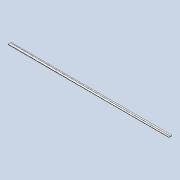
# Autodesk Inventor part: HTD 3M 780mm Open End Belt
Saved by Autodesk Inventor 2022 (Build 260153000, 153)
## iProperties
Created: 2021-10-10
Part Number: HTD 3M 780mm Open End Belt
Material: Generic
Document SubType Name: Modeling
Designer: Coy
Density: 1 g/cm^3
Appearance: Snow
Author: Coy
Autodesk Inventor part; units mm, degrees
(part 1 of 4)
ref_plane "YZ Plane" through (0, 0, 0) normal (1, 0, 0) x (0, 1, 0)
ref_plane "XZ Plane" through (0, 0, 0) normal (0, 1, 0) x (-1, 0, 0)
ref_plane "XY Plane" through (0, 0, 0) normal (0, 0, 1) x (1, 0, 0)
sketch "Sketch1" plane through (0, 0, 0) normal (0, 0, 1) x (1, 0, 0)
  line L0 (0, 2.4) -> (-3, 2.4)
  line L1 (0, 0) -> (-3, 0) construction
  line L2 (0, 2.4) -> (0, 0)
  line L3 (-3, 0) -> (-3, 2.4) construction
  arc A0 (-0.8878, 0.9525) -> (0, 0) centre (0, 0.89) ccw
  arc A1 (-3, 0) -> (-2.1122, 0.9525) centre (-3, 0.89) ccw
  line L4 (-1.1372, 1.22) -> (-1.8628, 1.22) construction
  line L5 (-1.5, 1.22) -> (-1.5, 0) construction
  line L6 (-1.8628, 1.22) -> (-1.1372, 1.22)
  arc A2 (-1.8628, 1.22) -> (-2.1122, 0.9525) centre (-1.8628, 0.97) ccw
  arc A3 (-0.8878, 0.9525) -> (-1.1372, 1.22) centre (-1.1372, 0.97) ccw
  line L7 (-6, 2.4) -> (-3, 2.4)
  line L8 (-6, 0) -> (-3, 0) construction
  line L9 (-6, 2.4) -> (-6, 0) construction
  arc A4 (-6, 0) -> (-5.1122, 0.9525) centre (-6, 0.89) ccw
  arc A5 (-3.8878, 0.9525) -> (-3, 0) centre (-3, 0.89) ccw
  line L10 (-4.8628, 1.22) -> (-4.1372, 1.22) construction
  line L11 (-4.5, 1.22) -> (-4.5, 0) construction
  line L12 (-4.1372, 1.22) -> (-4.8628, 1.22)
  arc A6 (-3.8878, 0.9525) -> (-4.1372, 1.22) centre (-4.1372, 0.97) ccw
  arc A7 (-4.8628, 1.22) -> (-5.1122, 0.9525) centre (-4.8628, 0.97) ccw
  line L13 (-12, 2.4) -> (-9, 2.4)
  line L14 (-12, 0) -> (-9, 0) construction
  line L15 (-12, 2.4) -> (-12, 0) construction
  line L16 (-9, 0) -> (-9, 2.4) construction
  arc A8 (-12, 0) -> (-11.1122, 0.9525) centre (-12, 0.89) ccw
  arc A9 (-9.8878, 0.9525) -> (-9, 0) centre (-9, 0.89) ccw
  line L17 (-10.8628, 1.22) -> (-10.1372, 1.22) construction
  line L18 (-10.5, 1.22) -> (-10.5, 0) construction
  line L19 (-10.1372, 1.22) -> (-10.8628, 1.22)
  arc A10 (-9.8878, 0.9525) -> (-10.1372, 1.22) centre (-10.1372, 0.97) ccw
  arc A11 (-10.8628, 1.22) -> (-11.1122, 0.9525) centre (-10.8628, 0.97) ccw
  line L20 (-6, 2.4) -> (-9, 2.4)
  line L21 (-6, 0) -> (-9, 0) construction
  arc A12 (-6.8878, 0.9525) -> (-6, 0) centre (-6, 0.89) ccw
  arc A13 (-9, 0) -> (-8.1122, 0.9525) centre (-9, 0.89) ccw
  line L22 (-7.1372, 1.22) -> (-7.8628, 1.22) construction
  line L23 (-7.5, 1.22) -> (-7.5, 0) construction
  line L24 (-7.8628, 1.22) -> (-7.1372, 1.22)
  arc A14 (-7.8628, 1.22) -> (-8.1122, 0.9525) centre (-7.8628, 0.97) ccw
  arc A15 (-6.8878, 0.9525) -> (-7.1372, 1.22) centre (-7.1372, 0.97) ccw
  line L25 (-24, 2.4) -> (-21, 2.4)
  line L26 (-24, 0) -> (-21, 0) construction
  line L27 (-24, 2.4) -> (-24, 0) construction
  line L28 (-21, 0) -> (-21, 2.4) construction
  arc A16 (-24, 0) -> (-23.1122, 0.9525) centre (-24, 0.89) ccw
  arc A17 (-21.8878, 0.9525) -> (-21, 0) centre (-21, 0.89) ccw
  line L29 (-22.8628, 1.22) -> (-22.1372, 1.22) construction
  line L30 (-22.5, 1.22) -> (-22.5, 0) construction
  line L31 (-22.1372, 1.22) -> (-22.8628, 1.22)
  arc A18 (-21.8878, 0.9525) -> (-22.1372, 1.22) centre (-22.1372, 0.97) ccw
  arc A19 (-22.8628, 1.22) -> (-23.1122, 0.9525) centre (-22.8628, 0.97) ccw
  line L32 (-18, 2.4) -> (-21, 2.4)
  line L33 (-18, 0) -> (-21, 0) construction
  line L34 (-18, 2.4) -> (-18, 0) construction
  arc A20 (-18.8878, 0.9525) -> (-18, 0) centre (-18, 0.89) ccw
  arc A21 (-21, 0) -> (-20.1122, 0.9525) centre (-21, 0.89) ccw
  line L35 (-19.1372, 1.22) -> (-19.8628, 1.22) construction
  line L36 (-19.5, 1.22) -> (-19.5, 0) construction
  line L37 (-19.8628, 1.22) -> (-19.1372, 1.22)
  arc A22 (-19.8628, 1.22) -> (-20.1122, 0.9525) centre (-19.8628, 0.97) ccw
  arc A23 (-18.8878, 0.9525) -> (-19.1372, 1.22) centre (-19.1372, 0.97) ccw
  line L38 (-15, 0) -> (-15, 2.4) construction
  arc A24 (-15.8878, 0.9525) -> (-15, 0) centre (-15, 0.89) ccw
  arc A25 (-15.8878, 0.9525) -> (-16.1372, 1.22) centre (-16.1372, 0.97) ccw
  line L39 (-16.5, 1.22) -> (-16.5, 0) construction
  line L40 (-16.8628, 1.22) -> (-16.1372, 1.22) construction
  line L41 (-16.1372, 1.22) -> (-16.8628, 1.22)
  arc A26 (-16.8628, 1.22) -> (-17.1122, 0.9525) centre (-16.8628, 0.97) ccw
  line L42 (-18, 0) -> (-15, 0) construction
  line L43 (-18, 2.4) -> (-15, 2.4)
  arc A27 (-18, 0) -> (-17.1122, 0.9525) centre (-18, 0.89) ccw
  line L44 (-12, 2.4) -> (-15, 2.4)
  line L45 (-12, 0) -> (-15, 0) construction
  arc A28 (-12.8878, 0.9525) -> (-12, 0) centre (-12, 0.89) ccw
  arc A29 (-15, 0) -> (-14.1122, 0.9525) centre (-15, 0.89) ccw
  line L46 (-13.1372, 1.22) -> (-13.8628, 1.22) construction
  arc A30 (-13.8628, 1.22) -> (-14.1122, 0.9525) centre (-13.8628, 0.97) ccw
  line L47 (-13.5, 1.22) -> (-13.5, 0) construction
  line L48 (-13.8628, 1.22) -> (-13.1372, 1.22)
  arc A31 (-12.8878, 0.9525) -> (-13.1372, 1.22) centre (-13.1372, 0.97) ccw
  line L49 (-48, 2.4) -> (-45, 2.4)
  line L50 (-48, 0) -> (-45, 0) construction
  line L51 (-48, 2.4) -> (-48, 0) construction
  line L52 (-45, 0) -> (-45, 2.4) construction
  arc A32 (-48, 0) -> (-47.1122, 0.9525) centre (-48, 0.89) ccw
  arc A33 (-45.8878, 0.9525) -> (-45, 0) centre (-45, 0.89) ccw
  line L53 (-46.8628, 1.22) -> (-46.1372, 1.22) construction
  line L54 (-46.5, 1.22) -> (-46.5, 0) construction
  line L55 (-46.1372, 1.22) -> (-46.8628, 1.22)
  arc A34 (-45.8878, 0.9525) -> (-46.1372, 1.22) centre (-46.1372, 0.97) ccw
  arc A35 (-46.8628, 1.22) -> (-47.1122, 0.9525) centre (-46.8628, 0.97) ccw
  line L56 (-42, 2.4) -> (-45, 2.4)
  line L57 (-42, 0) -> (-45, 0) construction
  line L58 (-42, 2.4) -> (-42, 0) construction
  arc A36 (-42.8878, 0.9525) -> (-42, 0) centre (-42, 0.89) ccw
  arc A37 (-45, 0) -> (-44.1122, 0.9525) centre (-45, 0.89) ccw
  line L59 (-43.1372, 1.22) -> (-43.8628, 1.22) construction
  line L60 (-43.5, 1.22) -> (-43.5, 0) construction
  line L61 (-43.8628, 1.22) -> (-43.1372, 1.22)
  arc A38 (-43.8628, 1.22) -> (-44.1122, 0.9525) centre (-43.8628, 0.97) ccw
  arc A39 (-42.8878, 0.9525) -> (-43.1372, 1.22) centre (-43.1372, 0.97) ccw
  line L62 (-39, 0) -> (-39, 2.4) construction
  arc A40 (-39.8878, 0.9525) -> (-39, 0) centre (-39, 0.89) ccw
  arc A41 (-39.8878, 0.9525) -> (-40.1372, 1.22) centre (-40.1372, 0.97) ccw
  line L63 (-40.5, 1.22) -> (-40.5, 0) construction
  line L64 (-40.8628, 1.22) -> (-40.1372, 1.22) construction
  line L65 (-40.1372, 1.22) -> (-40.8628, 1.22)
  arc A42 (-40.8628, 1.22) -> (-41.1122, 0.9525) centre (-40.8628, 0.97) ccw
  line L66 (-42, 0) -> (-39, 0) construction
  line L67 (-42, 2.4) -> (-39, 2.4)
  arc A43 (-42, 0) -> (-41.1122, 0.9525) centre (-42, 0.89) ccw
  line L68 (-36, 2.4) -> (-39, 2.4)
  line L69 (-36, 0) -> (-39, 0) construction
  line L70 (-36, 2.4) -> (-36, 0) construction
  arc A44 (-36.8878, 0.9525) -> (-36, 0) centre (-36, 0.89) ccw
  arc A45 (-39, 0) -> (-38.1122, 0.9525) centre (-39, 0.89) ccw
  line L71 (-37.1372, 1.22) -> (-37.8628, 1.22) construction
  arc A46 (-37.8628, 1.22) -> (-38.1122, 0.9525) centre (-37.8628, 0.97) ccw
  line L72 (-37.5, 1.22) -> (-37.5, 0) construction
  line L73 (-37.8628, 1.22) -> (-37.1372, 1.22)
  arc A47 (-36.8878, 0.9525) -> (-37.1372, 1.22) centre (-37.1372, 0.97) ccw
  line L74 (-27, 0) -> (-27, 2.4) construction
  arc A48 (-27.8878, 0.9525) -> (-27, 0) centre (-27, 0.89) ccw
  arc A49 (-27.8878, 0.9525) -> (-28.1372, 1.22) centre (-28.1372, 0.97) ccw
  line L75 (-28.5, 1.22) -> (-28.5, 0) construction
  line L76 (-28.8628, 1.22) -> (-28.1372, 1.22) construction
  line L77 (-28.1372, 1.22) -> (-28.8628, 1.22)
  arc A50 (-28.8628, 1.22) -> (-29.1122, 0.9525) centre (-28.8628, 0.97) ccw
  line L78 (-30, 0) -> (-27, 0) construction
  line L79 (-30, 2.4) -> (-27, 2.4)
  arc A51 (-30, 0) -> (-29.1122, 0.9525) centre (-30, 0.89) ccw
  line L80 (-30, 2.4) -> (-30, 0) construction
  arc A52 (-30.8878, 0.9525) -> (-30, 0) centre (-30, 0.89) ccw
  arc A53 (-30.8878, 0.9525) -> (-31.1372, 1.22) centre (-31.1372, 0.97) ccw
  line L81 (-31.5, 1.22) -> (-31.5, 0) construction
  line L82 (-31.1372, 1.22) -> (-31.8628, 1.22) construction
  line L83 (-31.8628, 1.22) -> (-31.1372, 1.22)
  arc A54 (-31.8628, 1.22) -> (-32.1122, 0.9525) centre (-31.8628, 0.97) ccw
  line L84 (-30, 0) -> (-33, 0) construction
  line L85 (-30, 2.4) -> (-33, 2.4)
  arc A55 (-33, 0) -> (-32.1122, 0.9525) centre (-33, 0.89) ccw
  line L86 (-33, 0) -> (-33, 2.4) construction
  arc A56 (-33.8878, 0.9525) -> (-33, 0) centre (-33, 0.89) ccw
  arc A57 (-33.8878, 0.9525) -> (-34.1372, 1.22) centre (-34.1372, 0.97) ccw
  line L87 (-34.5, 1.22) -> (-34.5, 0) construction
  line L88 (-34.8628, 1.22) -> (-34.1372, 1.22) construction
  line L89 (-34.1372, 1.22) -> (-34.8628, 1.22)
  arc A58 (-34.8628, 1.22) -> (-35.1122, 0.9525) centre (-34.8628, 0.97) ccw
  line L90 (-36, 2.4) -> (-33, 2.4)
  line L91 (-36, 0) -> (-33, 0) construction
  arc A59 (-36, 0) -> (-35.1122, 0.9525) centre (-36, 0.89) ccw
  line L92 (-24, 2.4) -> (-27, 2.4)
  line L93 (-24, 0) -> (-27, 0) construction
  arc A60 (-24.8878, 0.9525) -> (-24, 0) centre (-24, 0.89) ccw
  arc A61 (-27, 0) -> (-26.1122, 0.9525) centre (-27, 0.89) ccw
  arc A62 (-25.8628, 1.22) -> (-26.1122, 0.9525) centre (-25.8628, 0.97) ccw
  line L94 (-25.5, 1.22) -> (-25.5, 0) construction
  line L95 (-25.1372, 1.22) -> (-25.8628, 1.22) construction
  line L96 (-25.8628, 1.22) -> (-25.1372, 1.22)
  arc A63 (-24.8878, 0.9525) -> (-25.1372, 1.22) centre (-25.1372, 0.97) ccw
  line L97 (-96, 2.4) -> (-93, 2.4)
  line L98 (-96, 0) -> (-93, 0) construction
  line L99 (-96, 2.4) -> (-96, 0) construction
  line L100 (-93, 0) -> (-93, 2.4) construction
  arc A64 (-96, 0) -> (-95.1122, 0.9525) centre (-96, 0.89) ccw
  arc A65 (-93.8878, 0.9525) -> (-93, 0) centre (-93, 0.89) ccw
  line L101 (-94.8628, 1.22) -> (-94.1372, 1.22) construction
  line L102 (-94.5, 1.22) -> (-94.5, 0) construction
  line L103 (-94.1372, 1.22) -> (-94.8628, 1.22)
  arc A66 (-93.8878, 0.9525) -> (-94.1372, 1.22) centre (-94.1372, 0.97) ccw
  arc A67 (-94.8628, 1.22) -> (-95.1122, 0.9525) centre (-94.8628, 0.97) ccw
  line L104 (-90, 2.4) -> (-93, 2.4)
  line L105 (-90, 0) -> (-93, 0) construction
  line L106 (-90, 2.4) -> (-90, 0) construction
  arc A68 (-90.8878, 0.9525) -> (-90, 0) centre (-90, 0.89) ccw
  arc A69 (-93, 0) -> (-92.1122, 0.9525) centre (-93, 0.89) ccw
  line L107 (-91.1372, 1.22) -> (-91.8628, 1.22) construction
  line L108 (-91.5, 1.22) -> (-91.5, 0) construction
  line L109 (-91.8628, 1.22) -> (-91.1372, 1.22)
  arc A70 (-91.8628, 1.22) -> (-92.1122, 0.9525) centre (-91.8628, 0.97) ccw
  arc A71 (-90.8878, 0.9525) -> (-91.1372, 1.22) centre (-91.1372, 0.97) ccw
  line L110 (-87, 0) -> (-87, 2.4) construction
  arc A72 (-87.8878, 0.9525) -> (-87, 0) centre (-87, 0.89) ccw
  arc A73 (-87.8878, 0.9525) -> (-88.1372, 1.22) centre (-88.1372, 0.97) ccw
  line L111 (-88.5, 1.22) -> (-88.5, 0) construction
  line L112 (-88.8628, 1.22) -> (-88.1372, 1.22) construction
  line L113 (-88.1372, 1.22) -> (-88.8628, 1.22)
  arc A74 (-88.8628, 1.22) -> (-89.1122, 0.9525) centre (-88.8628, 0.97) ccw
  line L114 (-90, 0) -> (-87, 0) construction
  line L115 (-90, 2.4) -> (-87, 2.4)
  arc A75 (-90, 0) -> (-89.1122, 0.9525) centre (-90, 0.89) ccw
  line L116 (-84, 2.4) -> (-87, 2.4)
  line L117 (-84, 0) -> (-87, 0) construction
  line L118 (-84, 2.4) -> (-84, 0) construction
  arc A76 (-84.8878, 0.9525) -> (-84, 0) centre (-84, 0.89) ccw
  arc A77 (-87, 0) -> (-86.1122, 0.9525) centre (-87, 0.89) ccw
  line L119 (-85.1372, 1.22) -> (-85.8628, 1.22) construction
  arc A78 (-85.8628, 1.22) -> (-86.1122, 0.9525) centre (-85.8628, 0.97) ccw
  line L120 (-85.5, 1.22) -> (-85.5, 0) construction
  line L121 (-85.8628, 1.22) -> (-85.1372, 1.22)
  arc A79 (-84.8878, 0.9525) -> (-85.1372, 1.22) centre (-85.1372, 0.97) ccw
  line L122 (-75, 0) -> (-75, 2.4) construction
  arc A80 (-75.8878, 0.9525) -> (-75, 0) centre (-75, 0.89) ccw
  arc A81 (-75.8878, 0.9525) -> (-76.1372, 1.22) centre (-76.1372, 0.97) ccw
  line L123 (-76.5, 1.22) -> (-76.5, 0) construction
  line L124 (-76.8628, 1.22) -> (-76.1372, 1.22) construction
  line L125 (-76.1372, 1.22) -> (-76.8628, 1.22)
  arc A82 (-76.8628, 1.22) -> (-77.1122, 0.9525) centre (-76.8628, 0.97) ccw
  line L126 (-78, 0) -> (-75, 0) construction
  line L127 (-78, 2.4) -> (-75, 2.4)
  arc A83 (-78, 0) -> (-77.1122, 0.9525) centre (-78, 0.89) ccw
  line L128 (-78, 2.4) -> (-78, 0) construction
  arc A84 (-78.8878, 0.9525) -> (-78, 0) centre (-78, 0.89) ccw
  arc A85 (-78.8878, 0.9525) -> (-79.1372, 1.22) centre (-79.1372, 0.97) ccw
  line L129 (-79.5, 1.22) -> (-79.5, 0) construction
  line L130 (-79.1372, 1.22) -> (-79.8628, 1.22) construction
  line L131 (-79.8628, 1.22) -> (-79.1372, 1.22)
  arc A86 (-79.8628, 1.22) -> (-80.1122, 0.9525) centre (-79.8628, 0.97) ccw
  line L132 (-78, 0) -> (-81, 0) construction
  line L133 (-78, 2.4) -> (-81, 2.4)
  arc A87 (-81, 0) -> (-80.1122, 0.9525) centre (-81, 0.89) ccw
  line L134 (-81, 0) -> (-81, 2.4) construction
  arc A88 (-81.8878, 0.9525) -> (-81, 0) centre (-81, 0.89) ccw
  arc A89 (-81.8878, 0.9525) -> (-82.1372, 1.22) centre (-82.1372, 0.97) ccw
  line L135 (-82.5, 1.22) -> (-82.5, 0) construction
  line L136 (-82.8628, 1.22) -> (-82.1372, 1.22) construction
  line L137 (-82.1372, 1.22) -> (-82.8628, 1.22)
  arc A90 (-82.8628, 1.22) -> (-83.1122, 0.9525) centre (-82.8628, 0.97) ccw
  line L138 (-84, 2.4) -> (-81, 2.4)
  line L139 (-84, 0) -> (-81, 0) construction
  arc A91 (-84, 0) -> (-83.1122, 0.9525) centre (-84, 0.89) ccw
  line L140 (-72, 2.4) -> (-75, 2.4)
  line L141 (-72, 0) -> (-75, 0) construction
  line L142 (-72, 2.4) -> (-72, 0) construction
  arc A92 (-72.8878, 0.9525) -> (-72, 0) centre (-72, 0.89) ccw
  arc A93 (-75, 0) -> (-74.1122, 0.9525) centre (-75, 0.89) ccw
  arc A94 (-73.8628, 1.22) -> (-74.1122, 0.9525) centre (-73.8628, 0.97) ccw
  line L143 (-73.5, 1.22) -> (-73.5, 0) construction
  line L144 (-73.1372, 1.22) -> (-73.8628, 1.22) construction
  line L145 (-73.8628, 1.22) -> (-73.1372, 1.22)
  arc A95 (-72.8878, 0.9525) -> (-73.1372, 1.22) centre (-73.1372, 0.97) ccw
  line L146 (-48, 2.4) -> (-51, 2.4)
  line L147 (-48, 0) -> (-51, 0) construction
  arc A96 (-48.8878, 0.9525) -> (-48, 0) centre (-48, 0.89) ccw
  arc A97 (-51, 0) -> (-50.1122, 0.9525) centre (-51, 0.89) ccw
  line L148 (-49.1372, 1.22) -> (-49.8628, 1.22) construction
  arc A98 (-49.8628, 1.22) -> (-50.1122, 0.9525) centre (-49.8628, 0.97) ccw
  line L149 (-49.5, 1.22) -> (-49.5, 0) construction
  line L150 (-49.8628, 1.22) -> (-49.1372, 1.22)
  arc A99 (-48.8878, 0.9525) -> (-49.1372, 1.22) centre (-49.1372, 0.97) ccw
  line L151 (-51, 0) -> (-51, 2.4) construction
  arc A100 (-51.8878, 0.9525) -> (-51, 0) centre (-51, 0.89) ccw
  arc A101 (-51.8878, 0.9525) -> (-52.1372, 1.22) centre (-52.1372, 0.97) ccw
  line L152 (-52.5, 1.22) -> (-52.5, 0) construction
  line L153 (-52.8628, 1.22) -> (-52.1372, 1.22) construction
  line L154 (-52.1372, 1.22) -> (-52.8628, 1.22)
  arc A102 (-52.8628, 1.22) -> (-53.1122, 0.9525) centre (-52.8628, 0.97) ccw
  line L155 (-54, 0) -> (-51, 0) construction
  arc A103 (-54, 0) -> (-53.1122, 0.9525) centre (-54, 0.89) ccw
  line L156 (-54, 2.4) -> (-51, 2.4)
  line L157 (-54, 2.4) -> (-54, 0) construction
  arc A104 (-54.8878, 0.9525) -> (-54, 0) centre (-54, 0.89) ccw
  arc A105 (-54.8878, 0.9525) -> (-55.1372, 1.22) centre (-55.1372, 0.97) ccw
  line L158 (-55.5, 1.22) -> (-55.5, 0) construction
  line L159 (-55.1372, 1.22) -> (-55.8628, 1.22) construction
  line L160 (-55.8628, 1.22) -> (-55.1372, 1.22)
  arc A106 (-55.8628, 1.22) -> (-56.1122, 0.9525) centre (-55.8628, 0.97) ccw
  line L161 (-54, 0) -> (-57, 0) construction
  line L162 (-54, 2.4) -> (-57, 2.4)
  line L163 (-57, 0) -> (-57, 2.4) construction
  arc A107 (-57, 0) -> (-56.1122, 0.9525) centre (-57, 0.89) ccw
  arc A108 (-57.8878, 0.9525) -> (-57, 0) centre (-57, 0.89) ccw
  arc A109 (-57.8878, 0.9525) -> (-58.1372, 1.22) centre (-58.1372, 0.97) ccw
  line L164 (-58.5, 1.22) -> (-58.5, 0) construction
  line L165 (-58.8628, 1.22) -> (-58.1372, 1.22) construction
  line L166 (-58.1372, 1.22) -> (-58.8628, 1.22)
  arc A110 (-58.8628, 1.22) -> (-59.1122, 0.9525) centre (-58.8628, 0.97) ccw
  line L167 (-60, 0) -> (-57, 0) construction
  arc A111 (-60, 0) -> (-59.1122, 0.9525) centre (-60, 0.89) ccw
  line L168 (-60, 2.4) -> (-57, 2.4)
  line L169 (-69, 0) -> (-69, 2.4) construction
  arc A112 (-69, 0) -> (-68.1122, 0.9525) centre (-69, 0.89) ccw
  arc A113 (-67.8628, 1.22) -> (-68.1122, 0.9525) centre (-67.8628, 0.97) ccw
  line L170 (-67.5, 1.22) -> (-67.5, 0) construction
  line L171 (-66, 2.4) -> (-66, 0) construction
  arc A114 (-66.8878, 0.9525) -> (-66, 0) centre (-66, 0.89) ccw
  arc A115 (-66.8878, 0.9525) -> (-67.1372, 1.22) centre (-67.1372, 0.97) ccw
  line L172 (-67.1372, 1.22) -> (-67.8628, 1.22) construction
  line L173 (-66, 2.4) -> (-69, 2.4)
  line L174 (-66, 0) -> (-69, 0) construction
  line L175 (-67.8628, 1.22) -> (-67.1372, 1.22)
  arc A116 (-66, 0) -> (-65.1122, 0.9525) centre (-66, 0.89) ccw
  arc A117 (-64.8628, 1.22) -> (-65.1122, 0.9525) centre (-64.8628, 0.97) ccw
  line L176 (-64.5, 1.22) -> (-64.5, 0) construction
  line L177 (-64.8628, 1.22) -> (-64.1372, 1.22) construction
  line L178 (-64.1372, 1.22) -> (-64.8628, 1.22)
  arc A118 (-63.8878, 0.9525) -> (-64.1372, 1.22) centre (-64.1372, 0.97) ccw
  line L179 (-66, 0) -> (-63, 0) construction
  line L180 (-66, 2.4) -> (-63, 2.4)
  arc A119 (-63.8878, 0.9525) -> (-63, 0) centre (-63, 0.89) ccw
  line L181 (-63, 0) -> (-63, 2.4) construction
  line L182 (-60, 2.4) -> (-60, 0) construction
  arc A120 (-60.8878, 0.9525) -> (-60, 0) centre (-60, 0.89) ccw
  arc A121 (-60.8878, 0.9525) -> (-61.1372, 1.22) centre (-61.1372, 0.97) ccw
  line L183 (-61.5, 1.22) -> (-61.5, 0) construction
  line L184 (-61.1372, 1.22) -> (-61.8628, 1.22) construction
  line L185 (-61.8628, 1.22) -> (-61.1372, 1.22)
  line L186 (-60, 2.4) -> (-63, 2.4)
  line L187 (-60, 0) -> (-63, 0) construction
  arc A122 (-63, 0) -> (-62.1122, 0.9525) centre (-63, 0.89) ccw
  arc A123 (-61.8628, 1.22) -> (-62.1122, 0.9525) centre (-61.8628, 0.97) ccw
  arc A124 (-69.8878, 0.9525) -> (-69, 0) centre (-69, 0.89) ccw
  arc A125 (-69.8878, 0.9525) -> (-70.1372, 1.22) centre (-70.1372, 0.97) ccw
  line L188 (-70.5, 1.22) -> (-70.5, 0) construction
  line L189 (-70.8628, 1.22) -> (-70.1372, 1.22) construction
  line L190 (-70.1372, 1.22) -> (-70.8628, 1.22)
  arc A126 (-70.8628, 1.22) -> (-71.1122, 0.9525) centre (-70.8628, 0.97) ccw
  line L191 (-72, 0) -> (-69, 0) construction
  line L192 (-72, 2.4) -> (-69, 2.4)
  arc A127 (-72, 0) -> (-71.1122, 0.9525) centre (-72, 0.89) ccw
  line L193 (-192, 2.4) -> (-189, 2.4)
  line L194 (-192, 0) -> (-189, 0) construction
  line L195 (-192, 2.4) -> (-192, 0)
  line L196 (-189, 0) -> (-189, 2.4) construction
  arc A128 (-192, 0) -> (-191.1122, 0.9525) centre (-192, 0.89) ccw
  arc A129 (-189.8878, 0.9525) -> (-189, 0) centre (-189, 0.89) ccw
  line L197 (-190.8628, 1.22) -> (-190.1372, 1.22) construction
  line L198 (-190.5, 1.22) -> (-190.5, 0) construction
  line L199 (-190.1372, 1.22) -> (-190.8628, 1.22)
  arc A130 (-189.8878, 0.9525) -> (-190.1372, 1.22) centre (-190.1372, 0.97) ccw
  arc A131 (-190.8628, 1.22) -> (-191.1122, 0.9525) centre (-190.8628, 0.97) ccw
  line L200 (-186, 2.4) -> (-189, 2.4)
  line L201 (-186, 0) -> (-189, 0) construction
  line L202 (-186, 2.4) -> (-186, 0) construction
  arc A132 (-186.8878, 0.9525) -> (-186, 0) centre (-186, 0.89) ccw
  arc A133 (-189, 0) -> (-188.1122, 0.9525) centre (-189, 0.89) ccw
  line L203 (-187.1372, 1.22) -> (-187.8628, 1.22) construction
  line L204 (-187.5, 1.22) -> (-187.5, 0) construction
  line L205 (-187.8628, 1.22) -> (-187.1372, 1.22)
  arc A134 (-187.8628, 1.22) -> (-188.1122, 0.9525) centre (-187.8628, 0.97) ccw
  arc A135 (-186.8878, 0.9525) -> (-187.1372, 1.22) centre (-187.1372, 0.97) ccw
  line L206 (-183, 0) -> (-183, 2.4) construction
  arc A136 (-183.8878, 0.9525) -> (-183, 0) centre (-183, 0.89) ccw
  arc A137 (-183.8878, 0.9525) -> (-184.1372, 1.22) centre (-184.1372, 0.97) ccw
  line L207 (-184.5, 1.22) -> (-184.5, 0) construction
  line L208 (-184.8628, 1.22) -> (-184.1372, 1.22) construction
  line L209 (-184.1372, 1.22) -> (-184.8628, 1.22)
  arc A138 (-184.8628, 1.22) -> (-185.1122, 0.9525) centre (-184.8628, 0.97) ccw
  line L210 (-186, 0) -> (-183, 0) construction
  line L211 (-186, 2.4) -> (-183, 2.4)
  arc A139 (-186, 0) -> (-185.1122, 0.9525) centre (-186, 0.89) ccw
  line L212 (-180, 2.4) -> (-183, 2.4)
  line L213 (-180, 0) -> (-183, 0) construction
  line L214 (-180, 2.4) -> (-180, 0) construction
  arc A140 (-180.8878, 0.9525) -> (-180, 0) centre (-180, 0.89) ccw
  arc A141 (-183, 0) -> (-182.1122, 0.9525) centre (-183, 0.89) ccw
  line L215 (-181.1372, 1.22) -> (-181.8628, 1.22) construction
  arc A142 (-181.8628, 1.22) -> (-182.1122, 0.9525) centre (-181.8628, 0.97) ccw
  line L216 (-181.5, 1.22) -> (-181.5, 0) construction
  line L217 (-181.8628, 1.22) -> (-181.1372, 1.22)
  arc A143 (-180.8878, 0.9525) -> (-181.1372, 1.22) centre (-181.1372, 0.97) ccw
  line L218 (-171, 0) -> (-171, 2.4) construction
  arc A144 (-171.8878, 0.9525) -> (-171, 0) centre (-171, 0.89) ccw
  arc A145 (-171.8878, 0.9525) -> (-172.1372, 1.22) centre (-172.1372, 0.97) ccw
  line L219 (-172.5, 1.22) -> (-172.5, 0) construction
  line L220 (-172.8628, 1.22) -> (-172.1372, 1.22) construction
  line L221 (-172.1372, 1.22) -> (-172.8628, 1.22)
  arc A146 (-172.8628, 1.22) -> (-173.1122, 0.9525) centre (-172.8628, 0.97) ccw
  line L222 (-174, 0) -> (-171, 0) construction
  line L223 (-174, 2.4) -> (-171, 2.4)
  arc A147 (-174, 0) -> (-173.1122, 0.9525) centre (-174, 0.89) ccw
  line L224 (-174, 2.4) -> (-174, 0) construction
  arc A148 (-174.8878, 0.9525) -> (-174, 0) centre (-174, 0.89) ccw
  arc A149 (-174.8878, 0.9525) -> (-175.1372, 1.22) centre (-175.1372, 0.97) ccw
  line L225 (-175.5, 1.22) -> (-175.5, 0) construction
  line L226 (-175.1372, 1.22) -> (-175.8628, 1.22) construction
  line L227 (-175.8628, 1.22) -> (-175.1372, 1.22)
  arc A150 (-175.8628, 1.22) -> (-176.1122, 0.9525) centre (-175.8628, 0.97) ccw
  line L228 (-174, 0) -> (-177, 0) construction
  line L229 (-174, 2.4) -> (-177, 2.4)
  arc A151 (-177, 0) -> (-176.1122, 0.9525) centre (-177, 0.89) ccw
  line L230 (-177, 0) -> (-177, 2.4) construction
  arc A152 (-177.8878, 0.9525) -> (-177, 0) centre (-177, 0.89) ccw
  arc A153 (-177.8878, 0.9525) -> (-178.1372, 1.22) centre (-178.1372, 0.97) ccw
  line L231 (-178.5, 1.22) -> (-178.5, 0) construction
  line L232 (-178.8628, 1.22) -> (-178.1372, 1.22) construction
  line L233 (-178.1372, 1.22) -> (-178.8628, 1.22)
  arc A154 (-178.8628, 1.22) -> (-179.1122, 0.9525) centre (-178.8628, 0.97) ccw
  line L234 (-180, 2.4) -> (-177, 2.4)
  line L235 (-180, 0) -> (-177, 0) construction
  arc A155 (-180, 0) -> (-179.1122, 0.9525) centre (-180, 0.89) ccw
  line L236 (-168, 2.4) -> (-171, 2.4)
  line L237 (-168, 0) -> (-171, 0) construction
  line L238 (-168, 2.4) -> (-168, 0) construction
  arc A156 (-168.8878, 0.9525) -> (-168, 0) centre (-168, 0.89) ccw
  arc A157 (-171, 0) -> (-170.1122, 0.9525) centre (-171, 0.89) ccw
  arc A158 (-169.8628, 1.22) -> (-170.1122, 0.9525) centre (-169.8628, 0.97) ccw
  line L239 (-169.5, 1.22) -> (-169.5, 0) construction
  line L240 (-169.1372, 1.22) -> (-169.8628, 1.22) construction
  line L241 (-169.8628, 1.22) -> (-169.1372, 1.22)
  arc A159 (-168.8878, 0.9525) -> (-169.1372, 1.22) centre (-169.1372, 0.97) ccw
  line L242 (-144, 2.4) -> (-147, 2.4)
  line L243 (-144, 0) -> (-147, 0) construction
  line L244 (-144, 2.4) -> (-144, 0) construction
  arc A160 (-144.8878, 0.9525) -> (-144, 0) centre (-144, 0.89) ccw
  arc A161 (-147, 0) -> (-146.1122, 0.9525) centre (-147, 0.89) ccw
  line L245 (-145.1372, 1.22) -> (-145.8628, 1.22) construction
  arc A162 (-145.8628, 1.22) -> (-146.1122, 0.9525) centre (-145.8628, 0.97) ccw
  line L246 (-145.5, 1.22) -> (-145.5, 0) construction
  line L247 (-145.8628, 1.22) -> (-145.1372, 1.22)
  arc A163 (-144.8878, 0.9525) -> (-145.1372, 1.22) centre (-145.1372, 0.97) ccw
  line L248 (-147, 0) -> (-147, 2.4) construction
  arc A164 (-147.8878, 0.9525) -> (-147, 0) centre (-147, 0.89) ccw
  arc A165 (-147.8878, 0.9525) -> (-148.1372, 1.22) centre (-148.1372, 0.97) ccw
  line L249 (-148.5, 1.22) -> (-148.5, 0) construction
  line L250 (-148.8628, 1.22) -> (-148.1372, 1.22) construction
  line L251 (-148.1372, 1.22) -> (-148.8628, 1.22)
  arc A166 (-148.8628, 1.22) -> (-149.1122, 0.9525) centre (-148.8628, 0.97) ccw
  line L252 (-150, 0) -> (-147, 0) construction
  arc A167 (-150, 0) -> (-149.1122, 0.9525) centre (-150, 0.89) ccw
  line L253 (-150, 2.4) -> (-147, 2.4)
  line L254 (-150, 2.4) -> (-150, 0) construction
  arc A168 (-150.8878, 0.9525) -> (-150, 0) centre (-150, 0.89) ccw
  arc A169 (-150.8878, 0.9525) -> (-151.1372, 1.22) centre (-151.1372, 0.97) ccw
  line L255 (-151.5, 1.22) -> (-151.5, 0) construction
  line L256 (-151.1372, 1.22) -> (-151.8628, 1.22) construction
  line L257 (-151.8628, 1.22) -> (-151.1372, 1.22)
  arc A170 (-151.8628, 1.22) -> (-152.1122, 0.9525) centre (-151.8628, 0.97) ccw
  line L258 (-150, 0) -> (-153, 0) construction
  line L259 (-150, 2.4) -> (-153, 2.4)
  line L260 (-153, 0) -> (-153, 2.4) construction
  arc A171 (-153, 0) -> (-152.1122, 0.9525) centre (-153, 0.89) ccw
  arc A172 (-153.8878, 0.9525) -> (-153, 0) centre (-153, 0.89) ccw
  arc A173 (-153.8878, 0.9525) -> (-154.1372, 1.22) centre (-154.1372, 0.97) ccw
  line L261 (-154.5, 1.22) -> (-154.5, 0) construction
  line L262 (-154.8628, 1.22) -> (-154.1372, 1.22) construction
  line L263 (-154.1372, 1.22) -> (-154.8628, 1.22)
  arc A174 (-154.8628, 1.22) -> (-155.1122, 0.9525) centre (-154.8628, 0.97) ccw
  line L264 (-156, 0) -> (-153, 0) construction
  arc A175 (-156, 0) -> (-155.1122, 0.9525) centre (-156, 0.89) ccw
  line L265 (-156, 2.4) -> (-153, 2.4)
  line L266 (-165, 0) -> (-165, 2.4) construction
  arc A176 (-165, 0) -> (-164.1122, 0.9525) centre (-165, 0.89) ccw
  arc A177 (-163.8628, 1.22) -> (-164.1122, 0.9525) centre (-163.8628, 0.97) ccw
  line L267 (-163.5, 1.22) -> (-163.5, 0) construction
  line L268 (-162, 2.4) -> (-162, 0) construction
  arc A178 (-162.8878, 0.9525) -> (-162, 0) centre (-162, 0.89) ccw
  arc A179 (-162.8878, 0.9525) -> (-163.1372, 1.22) centre (-163.1372, 0.97) ccw
  line L269 (-163.1372, 1.22) -> (-163.8628, 1.22) construction
  line L270 (-162, 2.4) -> (-165, 2.4)
  line L271 (-162, 0) -> (-165, 0) construction
  line L272 (-163.8628, 1.22) -> (-163.1372, 1.22)
  arc A180 (-162, 0) -> (-161.1122, 0.9525) centre (-162, 0.89) ccw
  arc A181 (-160.8628, 1.22) -> (-161.1122, 0.9525) centre (-160.8628, 0.97) ccw
  line L273 (-160.5, 1.22) -> (-160.5, 0) construction
  line L274 (-160.8628, 1.22) -> (-160.1372, 1.22) construction
  line L275 (-160.1372, 1.22) -> (-160.8628, 1.22)
  arc A182 (-159.8878, 0.9525) -> (-160.1372, 1.22) centre (-160.1372, 0.97) ccw
  line L276 (-162, 0) -> (-159, 0) construction
  line L277 (-162, 2.4) -> (-159, 2.4)
  arc A183 (-159.8878, 0.9525) -> (-159, 0) centre (-159, 0.89) ccw
  line L278 (-159, 0) -> (-159, 2.4) construction
  line L279 (-156, 2.4) -> (-156, 0) construction
  arc A184 (-156.8878, 0.9525) -> (-156, 0) centre (-156, 0.89) ccw
  arc A185 (-156.8878, 0.9525) -> (-157.1372, 1.22) centre (-157.1372, 0.97) ccw
  line L280 (-157.5, 1.22) -> (-157.5, 0) construction
  line L281 (-157.1372, 1.22) -> (-157.8628, 1.22) construction
  line L282 (-157.8628, 1.22) -> (-157.1372, 1.22)
  line L283 (-156, 2.4) -> (-159, 2.4)
  line L284 (-156, 0) -> (-159, 0) construction
  arc A186 (-159, 0) -> (-158.1122, 0.9525) centre (-159, 0.89) ccw
  arc A187 (-157.8628, 1.22) -> (-158.1122, 0.9525) centre (-157.8628, 0.97) ccw
  arc A188 (-165.8878, 0.9525) -> (-165, 0) centre (-165, 0.89) ccw
  arc A189 (-165.8878, 0.9525) -> (-166.1372, 1.22) centre (-166.1372, 0.97) ccw
  line L285 (-166.5, 1.22) -> (-166.5, 0) construction
  line L286 (-166.8628, 1.22) -> (-166.1372, 1.22) construction
  line L287 (-166.1372, 1.22) -> (-166.8628, 1.22)
  arc A190 (-166.8628, 1.22) -> (-167.1122, 0.9525) centre (-166.8628, 0.97) ccw
  line L288 (-168, 0) -> (-165, 0) construction
  line L289 (-168, 2.4) -> (-165, 2.4)
  arc A191 (-168, 0) -> (-167.1122, 0.9525) centre (-168, 0.89) ccw
  line L290 (-99, 0) -> (-99, 2.4) construction
  arc A192 (-99.8878, 0.9525) -> (-99, 0) centre (-99, 0.89) ccw
  arc A193 (-99.8878, 0.9525) -> (-100.1372, 1.22) centre (-100.1372, 0.97) ccw
  line L291 (-100.5, 1.22) -> (-100.5, 0) construction
  line L292 (-100.8628, 1.22) -> (-100.1372, 1.22) construction
  line L293 (-100.1372, 1.22) -> (-100.8628, 1.22)
  line L294 (-102, 0) -> (-99, 0) construction
  line L295 (-102, 2.4) -> (-99, 2.4)
  arc A194 (-102, 0) -> (-101.1122, 0.9525) centre (-102, 0.89) ccw
  arc A195 (-100.8628, 1.22) -> (-101.1122, 0.9525) centre (-100.8628, 0.97) ccw
  line L296 (-102, 2.4) -> (-102, 0) construction
  arc A196 (-102.8878, 0.9525) -> (-102, 0) centre (-102, 0.89) ccw
  arc A197 (-102.8878, 0.9525) -> (-103.1372, 1.22) centre (-103.1372, 0.97) ccw
  line L297 (-103.5, 1.22) -> (-103.5, 0) construction
  line L298 (-103.1372, 1.22) -> (-103.8628, 1.22) construction
  line L299 (-103.8628, 1.22) -> (-103.1372, 1.22)
  arc A198 (-103.8628, 1.22) -> (-104.1122, 0.9525) centre (-103.8628, 0.97) ccw
  line L300 (-102, 0) -> (-105, 0) construction
  line L301 (-102, 2.4) -> (-105, 2.4)
  arc A199 (-105, 0) -> (-104.1122, 0.9525) centre (-105, 0.89) ccw
  line L302 (-105, 0) -> (-105, 2.4) construction
  arc A200 (-105.8878, 0.9525) -> (-105, 0) centre (-105, 0.89) ccw
  arc A201 (-105.8878, 0.9525) -> (-106.1372, 1.22) centre (-106.1372, 0.97) ccw
  line L303 (-106.5, 1.22) -> (-106.5, 0) construction
  line L304 (-106.8628, 1.22) -> (-106.1372, 1.22) construction
  line L305 (-106.1372, 1.22) -> (-106.8628, 1.22)
  arc A202 (-106.8628, 1.22) -> (-107.1122, 0.9525) centre (-106.8628, 0.97) ccw
  line L306 (-108, 2.4) -> (-105, 2.4)
  line L307 (-108, 0) -> (-105, 0) construction
  arc A203 (-108, 0) -> (-107.1122, 0.9525) centre (-108, 0.89) ccw
  line L308 (-108, 2.4) -> (-108, 0) construction
  arc A204 (-108.8878, 0.9525) -> (-108, 0) centre (-108, 0.89) ccw
  arc A205 (-108.8878, 0.9525) -> (-109.1372, 1.22) centre (-109.1372, 0.97) ccw
  line L309 (-109.5, 1.22) -> (-109.5, 0) construction
  line L310 (-109.1372, 1.22) -> (-109.8628, 1.22) construction
  line L311 (-109.8628, 1.22) -> (-109.1372, 1.22)
  arc A206 (-109.8628, 1.22) -> (-110.1122, 0.9525) centre (-109.8628, 0.97) ccw
  line L312 (-108, 2.4) -> (-111, 2.4)
  line L313 (-108, 0) -> (-111, 0) construction
  arc A207 (-111, 0) -> (-110.1122, 0.9525) centre (-111, 0.89) ccw
  line L314 (-96, 2.4) -> (-99, 2.4)
  line L315 (-96, 0) -> (-99, 0) construction
  arc A208 (-96.8878, 0.9525) -> (-96, 0) centre (-96, 0.89) ccw
  arc A209 (-99, 0) -> (-98.1122, 0.9525) centre (-99, 0.89) ccw
  arc A210 (-97.8628, 1.22) -> (-98.1122, 0.9525) centre (-97.8628, 0.97) ccw
  line L316 (-97.5, 1.22) -> (-97.5, 0) construction
  line L317 (-97.1372, 1.22) -> (-97.8628, 1.22) construction
  line L318 (-97.8628, 1.22) -> (-97.1372, 1.22)
  arc A211 (-96.8878, 0.9525) -> (-97.1372, 1.22) centre (-97.1372, 0.97) ccw
  line L319 (-114, 2.4) -> (-114, 0) construction
  line L320 (-111, 0) -> (-111, 2.4) construction
  arc A212 (-111.8878, 0.9525) -> (-111, 0) centre (-111, 0.89) ccw
  arc A213 (-111.8878, 0.9525) -> (-112.1372, 1.22) centre (-112.1372, 0.97) ccw
  line L321 (-112.8628, 1.22) -> (-112.1372, 1.22) construction
  line L322 (-112.1372, 1.22) -> (-112.8628, 1.22)
  line L323 (-114, 2.4) -> (-111, 2.4)
  line L324 (-114, 0) -> (-111, 0) construction
  arc A214 (-112.8628, 1.22) -> (-113.1122, 0.9525) centre (-112.8628, 0.97) ccw
  line L325 (-117, 0) -> (-117, 2.4) construction
  arc A215 (-117.8878, 0.9525) -> (-118.1372, 1.22) centre (-118.1372, 0.97) ccw
  line L326 (-118.5, 1.22) -> (-118.5, 0) construction
  line L327 (-118.8628, 1.22) -> (-118.1372, 1.22) construction
  line L328 (-118.1372, 1.22) -> (-118.8628, 1.22)
  arc A216 (-118.8628, 1.22) -> (-119.1122, 0.9525) centre (-118.8628, 0.97) ccw
  line L329 (-120, 2.4) -> (-117, 2.4)
  line L330 (-120, 0) -> (-117, 0) construction
  arc A217 (-120, 0) -> (-119.1122, 0.9525) centre (-120, 0.89) ccw
  arc A218 (-117, 0) -> (-116.1122, 0.9525) centre (-117, 0.89) ccw
  arc A219 (-115.8628, 1.22) -> (-116.1122, 0.9525) centre (-115.8628, 0.97) ccw
  line L331 (-115.5, 1.22) -> (-115.5, 0) construction
  line L332 (-115.1372, 1.22) -> (-115.8628, 1.22) construction
  line L333 (-115.8628, 1.22) -> (-115.1372, 1.22)
  arc A220 (-114.8878, 0.9525) -> (-115.1372, 1.22) centre (-115.1372, 0.97) ccw
  line L334 (-114, 0) -> (-117, 0) construction
  line L335 (-114, 2.4) -> (-117, 2.4)
  arc A221 (-114.8878, 0.9525) -> (-114, 0) centre (-114, 0.89) ccw
  arc A222 (-114, 0) -> (-113.1122, 0.9525) centre (-114, 0.89) ccw
  line L336 (-112.5, 1.22) -> (-112.5, 0) construction
  arc A223 (-117.8878, 0.9525) -> (-117, 0) centre (-117, 0.89) ccw
  line L337 (-144, 2.4) -> (-141, 2.4)
  line L338 (-144, 0) -> (-141, 0) construction
  arc A224 (-144, 0) -> (-143.1122, 0.9525) centre (-144, 0.89) ccw
  arc A225 (-141.8878, 0.9525) -> (-141, 0) centre (-141, 0.89) ccw
  line L339 (-142.8628, 1.22) -> (-142.1372, 1.22) construction
  arc A226 (-141.8878, 0.9525) -> (-142.1372, 1.22) centre (-142.1372, 0.97) ccw
  line L340 (-142.1372, 1.22) -> (-142.8628, 1.22)
  arc A227 (-142.8628, 1.22) -> (-143.1122, 0.9525) centre (-142.8628, 0.97) ccw
  line L341 (-142.5, 1.22) -> (-142.5, 0) construction
  arc A228 (-141, 0) -> (-140.1122, 0.9525) centre (-141, 0.89) ccw
  arc A229 (-139.8628, 1.22) -> (-140.1122, 0.9525) centre (-139.8628, 0.97) ccw
  line L342 (-139.5, 1.22) -> (-139.5, 0) construction
  line L343 (-141, 0) -> (-141, 2.4) construction
  line L344 (-139.1372, 1.22) -> (-139.8628, 1.22) construction
  arc A230 (-138.8878, 0.9525) -> (-139.1372, 1.22) centre (-139.1372, 0.97) ccw
  line L345 (-138, 0) -> (-141, 0) construction
  line L346 (-138, 2.4) -> (-141, 2.4)
  arc A231 (-138.8878, 0.9525) -> (-138, 0) centre (-138, 0.89) ccw
  line L347 (-138, 2.4) -> (-138, 0) construction
  line L348 (-139.8628, 1.22) -> (-139.1372, 1.22)
  arc A232 (-138, 0) -> (-137.1122, 0.9525) centre (-138, 0.89) ccw
  arc A233 (-136.8628, 1.22) -> (-137.1122, 0.9525) centre (-136.8628, 0.97) ccw
  line L349 (-136.5, 1.22) -> (-136.5, 0) construction
  line L350 (-136.1372, 1.22) -> (-136.8628, 1.22)
  arc A234 (-135.8878, 0.9525) -> (-136.1372, 1.22) centre (-136.1372, 0.97) ccw
  line L351 (-138, 2.4) -> (-135, 2.4)
  line L352 (-138, 0) -> (-135, 0) construction
  line L353 (-135, 0) -> (-135, 2.4) construction
  arc A235 (-135.8878, 0.9525) -> (-135, 0) centre (-135, 0.89) ccw
  line L354 (-136.8628, 1.22) -> (-136.1372, 1.22) construction
  arc A236 (-135, 0) -> (-134.1122, 0.9525) centre (-135, 0.89) ccw
  arc A237 (-133.8628, 1.22) -> (-134.1122, 0.9525) centre (-133.8628, 0.97) ccw
  line L355 (-133.5, 1.22) -> (-133.5, 0) construction
  line L356 (-133.1372, 1.22) -> (-133.8628, 1.22) construction
  line L357 (-133.8628, 1.22) -> (-133.1372, 1.22)
  arc A238 (-132.8878, 0.9525) -> (-133.1372, 1.22) centre (-133.1372, 0.97) ccw
  line L358 (-132, 0) -> (-135, 0) construction
  line L359 (-132, 2.4) -> (-135, 2.4)
  line L360 (-132, 2.4) -> (-132, 0) construction
  arc A239 (-132.8878, 0.9525) -> (-132, 0) centre (-132, 0.89) ccw
  line L361 (-123, 0) -> (-123, 2.4) construction
  arc A240 (-123.8878, 0.9525) -> (-123, 0) centre (-123, 0.89) ccw
  arc A241 (-123.8878, 0.9525) -> (-124.1372, 1.22) centre (-124.1372, 0.97) ccw
  line L362 (-124.5, 1.22) -> (-124.5, 0) construction
  line L363 (-126, 2.4) -> (-126, 0) construction
  arc A242 (-126, 0) -> (-125.1122, 0.9525) centre (-126, 0.89) ccw
  arc A243 (-124.8628, 1.22) -> (-125.1122, 0.9525) centre (-124.8628, 0.97) ccw
  line L364 (-124.1372, 1.22) -> (-124.8628, 1.22)
  line L365 (-126, 0) -> (-123, 0) construction
  line L366 (-126, 2.4) -> (-123, 2.4)
  line L367 (-124.8628, 1.22) -> (-124.1372, 1.22) construction
  arc A244 (-126.8878, 0.9525) -> (-126, 0) centre (-126, 0.89) ccw
  arc A245 (-126.8878, 0.9525) -> (-127.1372, 1.22) centre (-127.1372, 0.97) ccw
  line L368 (-127.5, 1.22) -> (-127.5, 0) construction
  line L369 (-127.1372, 1.22) -> (-127.8628, 1.22) construction
  line L370 (-127.8628, 1.22) -> (-127.1372, 1.22)
  arc A246 (-127.8628, 1.22) -> (-128.1122, 0.9525) centre (-127.8628, 0.97) ccw
  line L371 (-126, 0) -> (-129, 0) construction
  line L372 (-126, 2.4) -> (-129, 2.4)
  line L373 (-129, 0) -> (-129, 2.4) construction
  arc A247 (-129, 0) -> (-128.1122, 0.9525) centre (-129, 0.89) ccw
  arc A248 (-132, 0) -> (-131.1122, 0.9525) centre (-132, 0.89) ccw
  arc A249 (-130.8628, 1.22) -> (-131.1122, 0.9525) centre (-130.8628, 0.97) ccw
  line L374 (-130.5, 1.22) -> (-130.5, 0) construction
  line L375 (-130.8628, 1.22) -> (-130.1372, 1.22) construction
  line L376 (-130.1372, 1.22) -> (-130.8628, 1.22)
  arc A250 (-129.8878, 0.9525) -> (-130.1372, 1.22) centre (-130.1372, 0.97) ccw
  line L377 (-132, 2.4) -> (-129, 2.4)
  line L378 (-132, 0) -> (-129, 0) construction
  arc A251 (-129.8878, 0.9525) -> (-129, 0) centre (-129, 0.89) ccw
  line L379 (-120, 2.4) -> (-120, 0) construction
  arc A252 (-120.8878, 0.9525) -> (-120, 0) centre (-120, 0.89) ccw
  arc A253 (-120.8878, 0.9525) -> (-121.1372, 1.22) centre (-121.1372, 0.97) ccw
  line L380 (-121.5, 1.22) -> (-121.5, 0) construction
  line L381 (-121.1372, 1.22) -> (-121.8628, 1.22) construction
  line L382 (-121.8628, 1.22) -> (-121.1372, 1.22)
  arc A254 (-121.8628, 1.22) -> (-122.1122, 0.9525) centre (-121.8628, 0.97) ccw
  line L383 (-120, 0) -> (-123, 0) construction
  arc A255 (-123, 0) -> (-122.1122, 0.9525) centre (-123, 0.89) ccw
  line L384 (-120, 2.4) -> (-123, 2.4)
  dimension "d0" = 3
  dimension "d1" = 2.4
  dimension "d2" = 1.78
  dimension "d4" = 1.78
  dimension "d5" = 1.22
  dimension "d6" = 0.25
  constraints: 770 end point, 725 symmetric about line, 512 point on circle, 256 centre point, 98 point on line, 5 tangent, 2 horizontal, 2 midpoint, 2 perpendicular, 1 equal radius, 1 parallel, 252 other
  measures "d0" distance of L0.start L0.end
  measures "d1" distance of L1.start L0.start
  measures "d2" diameter of A0
  measures "d4" diameter of A1
  measures "d5" distance from line of L1.start L4
  measures "d6" radius of A2
extrude "Extrusion1" add sketch "Sketch1" along normal blind 15